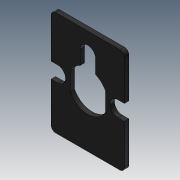
# Autodesk Inventor part: Quick Release Rubber Pad
Saved by Autodesk Inventor 2011 (Build 150239000, 239)
## iProperties
Created: 2012-11-06
Part Number: Quick Release Rubber Pad
Material: Rubber
Document SubType Name: Modeling
Designer: Lance
Mass: 2.16571 g
Surface Area: 28.2611 cm^2
Volume: 2.32872 cm^3
Density: 0.93 g/cm^3
Author: Lance
Autodesk Inventor part; units mm, degrees
ref_plane "YZ Plane" through (0, 0, 0) normal (1, 0, 0) x (0, 1, 0)
ref_plane "XZ Plane" through (0, 0, 0) normal (0, 1, 0) x (-1, 0, 0)
ref_plane "XY Plane" through (0, 0, 0) normal (0, 0, 1) x (1, 0, 0)
sketch "Sketch1" plane through (0, 0, 0) normal (0, 1, 0) x (-1, 0, 0)
  line L0 (16.5, -23.5) -> (-16.5, -23.5)
  line L1 (-16.5, -23.5) -> (-16.5, 23.5)
  line L2 (-16.5, 23.5) -> (16.5, 23.5)
  line L3 (16.5, 23.5) -> (16.5, -23.5)
  point P0 (0, 0)
  point P1 (16.5, 0)
  point P2 (0, -23.5)
  dimension "d0" = 33
  dimension "d1" = 47
  constraints: 8 end point, 2 midpoint, 2 parallel, 1 horizontal, 1 horizontal alignment, 1 perpendicular, 1 vertical alignment
  measures "d0" distance between parallel lines of L1 L3
  measures "d1" distance between parallel lines of L2 L0
extrude "Extrusion1" add sketch "Sketch1" along normal mid plane 2
sketch "Sketch2" plane through (0, 1, 0) normal (0, 1, 0) x (1, 0, 0)
  circle A0 centre (0, 0) radius 9
  line L0 (-8, -4.1231) -> (-8, 4.1231)
  line L1 (8, 4.1231) -> (8, -4.1231)
  line L2 (0, 32.9) -> (0, -32.9) projected
  dimension "d4" = 18
  dimension "d5" = 16
  constraints: 4 end point, 4 point on circle, 1 centre point, 1 coincident, 1 parallel, 1 vertical, 1 other
  measures "d4" diameter of A0
  measures "d5" distance between parallel lines of L1 L0
extrude "Extrusion2" cut sketch "Sketch2" against normal through all contours L1 A0 L2 | L2 A0 L0
sketch "Sketch3" plane through (0, 1, 0) normal (0, 1, 0) x (1, 0, 0)
  line L0 (-3.5, -8.2916) -> (-3.5, -14.5)
  arc A0 (-3.5, -14.5) -> (3.5, -14.5) centre (0, -14.5) ccw
  line L1 (3.5, -14.5) -> (3.5, -8.2916)
  line L2 (16.5, -3.5) -> (13.5, -3.5)
  arc A1 (13.5, 3.5) -> (13.5, -3.5) centre (13.5, 0) ccw
  line L3 (13.5, 3.5) -> (16.5, 3.5)
  line L4 (-16.5, 3.5) -> (-13.5, 3.5)
  arc A2 (-13.5, -3.5) -> (-13.5, 3.5) centre (-13.5, 0) ccw
  line L5 (-13.5, -3.5) -> (-16.5, -3.5)
  line L6 (8, 4.1231) -> (8, -4.1231) projected
  arc A3 (-8, -4.1231) -> (8, -4.1231) centre (0, 0) ccw projected
  line L7 (-8, -4.1231) -> (-8, 4.1231) projected
  arc A4 (8, 4.1231) -> (-8, 4.1231) centre (0, 0) ccw projected
  line L8 (16.5, 23.5) -> (16.5, -23.5) projected
  line L9 (-16.5, 23.5) -> (16.5, 23.5) projected
  line L10 (-16.5, -23.5) -> (-16.5, 23.5) projected
  line L11 (16.5, -23.5) -> (-16.5, -23.5) projected
  line L12 (-23.1, 0) -> (23.1, 0) projected
  line L13 (0, 32.9) -> (0, -32.9) projected
  dimension "d8" = 20
  dimension "d9" = 7
  dimension "d10" = 7
  dimension "d11" = 27
  constraints: 12 end point, 8 point on circle, 6 tangent, 4 equal length, 4 point on line, 3 centre point, 1 perpendicular, 1 vertical, 5 other
  measures "d9" distance between parallel lines of L3 L2
  measures "d10" distance between parallel lines of L1 L0
extrude "Extrusion3" cut sketch "Sketch3" against normal through all contours A3 L13 A0 L0 | A3 L1 A0 L13 | L12 L10 L4 A2 | A2 L5 L10 L12 | L12 L8 L2 A1 | A1 L3 L8 L12
fillet "Fillet1" radius 2 4 edges at (-16.5, 0, 23.5) (16.5, 0, 23.5) (16.5, 0, -23.5) (-16.5, 0, -23.5)
body "Solid1"
